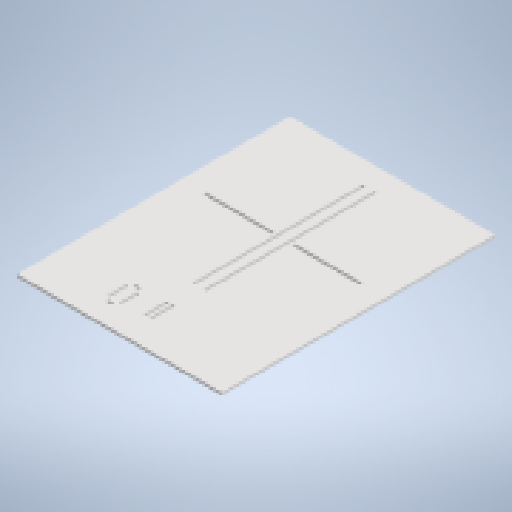
# Autodesk Inventor part: base
Saved by Autodesk Inventor 2023 (Build 270158000, 158)
## iProperties
Created: 2023-10-15
Part Number: base
Material: Generic
Document SubType Name: Modeling
Designer: Nate
Density: 1 g/cm^3
Appearance: Default
Author: Nate
Autodesk Inventor part; units mm, degrees
ref_plane "YZ Plane" through (0, 0, 0) normal (1, 0, 0) x (0, 1, 0)
ref_plane "XZ Plane" through (0, 0, 0) normal (0, 1, 0) x (-1, 0, 0)
ref_plane "XY Plane" through (0, 0, 0) normal (0, 0, 1) x (1, 0, 0)
sketch "Sketch1" plane through (0, 0, 0) normal (0, 1, 0) x (-1, 0, 0)
  line L0 (0, 0) -> (-457.2, 0)
  line L1 (-457.2, 0) -> (-457.2, -609.6)
  line L2 (-457.2, -609.6) -> (0, -609.6)
  line L3 (0, -609.6) -> (0, 0)
  line L4 (-212.725, -558.8) -> (-219.075, -558.8)
  line L5 (-219.075, -558.8) -> (-219.075, -177.8)
  line L6 (-219.075, -177.8) -> (-212.725, -177.8)
  line L7 (-212.725, -177.8) -> (-212.725, -558.8)
  line L8 (-238.125, -558.8) -> (-244.475, -558.8)
  line L9 (-244.475, -558.8) -> (-244.475, -177.8)
  line L10 (-244.475, -177.8) -> (-238.125, -177.8)
  line L11 (-238.125, -177.8) -> (-238.125, -558.8)
  line L12 (-53.975, -368.3) -> (-206.375, -368.3)
  line L13 (-206.375, -368.3) -> (-206.375, -361.95)
  line L14 (-206.375, -361.95) -> (-53.975, -361.95)
  line L15 (-53.975, -361.95) -> (-53.975, -368.3)
  line L16 (-250.825, -368.3) -> (-403.225, -368.3)
  line L17 (-403.225, -368.3) -> (-403.225, -361.95)
  line L18 (-403.225, -361.95) -> (-250.825, -361.95)
  line L19 (-250.825, -361.95) -> (-250.825, -368.3)
  line L20 (-219.075, -63.5) -> (-225.425, -63.5)
  line L21 (-225.425, -63.5) -> (-225.425, -114.3)
  line L22 (-225.425, -114.3) -> (-219.075, -114.3)
  line L23 (-219.075, -114.3) -> (-219.075, -63.5)
  line L24 (-231.775, -63.5) -> (-238.125, -63.5)
  line L25 (-238.125, -63.5) -> (-238.125, -114.3)
  line L26 (-238.125, -114.3) -> (-231.775, -114.3)
  line L27 (-231.775, -114.3) -> (-231.775, -63.5)
  line L28 (-148.2852, -105.5116) -> (-168.275, -105.5116)
  line L29 (-168.275, -105.5116) -> (-168.275, -52.07)
  line L30 (-168.275, -52.07) -> (-148.2852, -52.07)
  line L31 (-148.2852, -52.07) -> (-148.2852, -105.5116)
  line L32 (-151.9301, -105.5116) -> (-164.6301, -105.5116)
  line L33 (-164.6301, -105.5116) -> (-164.6301, -111.8616)
  line L34 (-164.6301, -111.8616) -> (-151.9301, -111.8616)
  line L35 (-151.9301, -111.8616) -> (-151.9301, -105.5116)
  line L36 (-151.9301, -52.07) -> (-164.6301, -52.07)
  line L37 (-164.6301, -52.07) -> (-164.6301, -45.72)
  line L38 (-164.6301, -45.72) -> (-151.9301, -45.72)
  line L39 (-151.9301, -45.72) -> (-151.9301, -52.07)
  line L40 (-148.2852, -99.1108) -> (-141.9352, -99.1108)
  line L41 (-141.9352, -99.1108) -> (-141.9352, -58.4708)
  line L42 (-141.9352, -58.4708) -> (-148.2852, -58.4708)
  line L43 (-148.2852, -58.4708) -> (-148.2852, -99.1108)
  line L44 (-168.275, -58.4708) -> (-174.625, -58.4708)
  line L45 (-174.625, -58.4708) -> (-174.625, -99.1108)
  line L46 (-174.625, -99.1108) -> (-168.275, -99.1108)
  line L47 (-168.275, -99.1108) -> (-168.275, -58.4708)
  point P0 (-215.9, -558.8)
  point P1 (-215.9, -177.8)
  point P2 (-241.3, -558.8)
  point P3 (-241.3, -177.8)
  point P4 (-212.725, -368.3)
  point P5 (-206.375, -365.125)
  point P6 (-250.825, -365.125)
  point P7 (-222.25, -63.5)
  point P8 (-158.2801, -105.5116)
  point P9 (-151.9301, -108.6866)
  point P10 (-151.9301, -48.895)
  point P11 (-145.1102, -99.1108)
  dimension "d0" = 457.2
  dimension "d1" = 609.6
  dimension "d2" = 6.35
  dimension "d3" = 6.35
  dimension "d4" = 381
  dimension "d5" = 381
  dimension "d6" = 50.8
  dimension "d7" = 50.8
  dimension "d8" = 19.05
  dimension "d9" = 212.725
  dimension "d10" = 152.4
  dimension "d11" = 6.35
  dimension "d12" = 241.3
  dimension "d13" = 6.35
  dimension "d14" = 152.4
  dimension "d15" = 6.35
  dimension "d16" = 6.35
  dimension "d17" = 241.3
  dimension "d18" = 6.35
  dimension "d19" = 50.8
  dimension "d20" = 6.35
  dimension "d21" = 50.8
  dimension "d22" = 6.35
  dimension "d23" = 219.075
  dimension "d24" = 19.9898
  dimension "d25" = 53.4416
  dimension "d26" = 50.8
  dimension "d27" = 63.5
  dimension "d29" = 105.5116
  dimension "d30" = 12.7
  dimension "d31" = 6.35
  dimension "d32" = 3.6449
  dimension "d33" = 12.7
  dimension "d34" = 6.35
  dimension "d35" = 3.6449
  dimension "d36" = 6.35
  dimension "d37" = 40.64
  dimension "d38" = 6.4008
  dimension "d39" = 6.35
  dimension "d40" = 40.64
  dimension "d41" = 6.4008
  constraints: 96 end point, 24 parallel, 12 horizontal, 12 midpoint, 12 perpendicular, 5 point on line
  measures "d0" distance of L2.end L1.end
  measures "d1" distance of L1.end L0.end
  measures "d2" distance of L5.end L6.end
  measures "d3" distance of L9.end L10.end
  measures "d4" distance of point (-215.9, -558.8) point (-215.9, -177.8)
  measures "d5" distance of point (-241.3, -558.8) point (-241.3, -177.8)
  measures "d6" distance from line of L2 point (-215.9, -558.8)
  measures "d7" distance between parallel lines of L2 L8
  measures "d8" distance between parallel lines of L11 L5
  measures "d9" distance between parallel lines of L7 L3
  measures "d10" distance of L13.end L14.end
  measures "d11" distance between parallel lines of L12 L14
  measures "d12" distance between parallel lines of L2 L12
  measures "d13" horizontal distance of point (-212.725, -368.3) point (-206.375, -365.125)
  measures "d14" distance of L17.end L18.end
  measures "d15" distance between parallel lines of L16 L18
  measures "d16" distance from line of L9 point (-250.825, -365.125)
  measures "d17" distance between parallel lines of L2 L16
  measures "d18" distance of L22.end L21.end
  measures "d19" distance of L21.end L20.end
  measures "d20" distance of L26.end L25.end
  measures "d21" distance of L25.end L24.end
  measures "d22" distance between parallel lines of L27 L21
  measures "d23" distance between parallel lines of L3 L23
  measures "d24" distance of L29.end L30.end
  measures "d25" distance of L28.end L29.end
  measures "d26" distance between parallel lines of L23 L29
  measures "d27" distance from line of L0 point (-222.25, -63.5)
  measures "d29" distance from line of L0 point (-158.28, -105.512)
  measures "d30" distance of L34.end L33.end
  measures "d31" distance between parallel lines of L34 L32
  measures "d32" distance from line of point (-151.93, -108.687) L31
  measures "d33" distance of L37.end L38.end
  measures "d34" distance of L36.end L37.end
  measures "d35" distance from line of L31 point (-151.93, -48.895)
  measures "d36" distance of L42.end L41.end
  measures "d37" distance of L41.end L40.end
  measures "d38" distance from line of L28 point (-145.11, -99.111)
  measures "d39" distance of L46.end L45.end
  measures "d40" distance between parallel lines of L46 L44
  measures "d41" distance between parallel lines of L28 L46
extrude "Extrusion1" add sketch "Sketch1" along normal blind 6.35 contours L3 L2 L1 L0 | L28 L29 L30 L31
body "Solid1"
